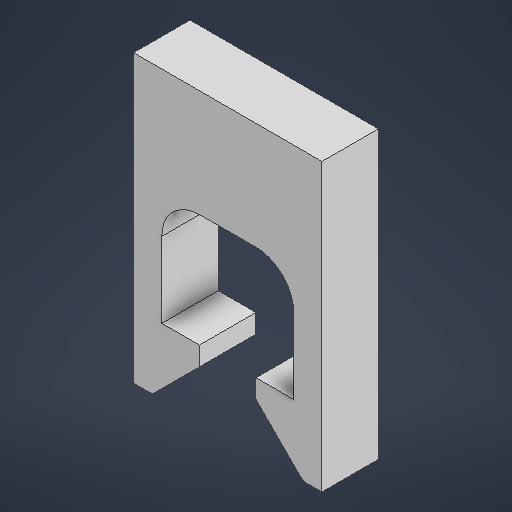
# Autodesk Inventor part: P_Wing_Mountingplate_pin
Saved by Autodesk Inventor 2026 (Build 300175000, 175)
## iProperties
Created: 2025-09-10
Part Number: P_Wing_Mountingplate_pin
Material: Generisch
Document SubType Name: Modeling
Designer: FAL
Density: 1 g/cm^3
Appearance: Vorgabe
Author: FAL
Autodesk Inventor part; units mm, degrees
ref_plane "YZ Plane" through (0, 0, 0) normal (1, 0, 0) x (0, 1, 0)
ref_plane "XZ Plane" through (0, 0, 0) normal (0, 1, 0) x (-1, 0, 0)
ref_plane "XY Plane" through (0, 0, 0) normal (0, 0, 1) x (1, 0, 0)
sketch "Skizze3" plane through (0, 0, 0) normal (0, 1, 0) x (-1, 0, 0)
  line L0 (3.5, 0) -> (3.5, -6)
  line L1 (3.5, -6) -> (1.5, -6)
  line L2 (1.5, -6) -> (1.5, -7)
  line L3 (1.5, -7) -> (4, -9.5)
  line L4 (4, -9.5) -> (5, -9.5)
  line L5 (5, -9.5) -> (5, 15)
  line L6 (5, 15) -> (0, 15)
  line L7 (0, 15) -> (0, 0)
  line L8 (0, 0) -> (3.5, 0)
  dimension "d11" = 1.5
  dimension "d12" = 6
  dimension "d13" = 1
  dimension "d14" = 1
  dimension "d15" = 45
  dimension "d16" = 2
  dimension "d17" = 5
  dimension "d18" = 15
  constraints: 18 end point, 4 perpendicular, 2 vertical, 1 coincident, 1 horizontal, 1 parallel
  measures "d11" distance between parallel lines of L0 L5
  measures "d12" distance between parallel lines of L8 L1
  measures "d13" distance of L1.end L2.end
  measures "d14" distance of L3.end L4.end
  measures "d15" angle of L0 L3
  measures "d16" distance between parallel lines of L0 L2
  measures "d17" distance between parallel lines of L7 L5
  measures "d18" distance between parallel lines of L8 L6
extrude "Extrusion2" add sketch "Skizze3" along normal blind 3
fillet "Rundung3" radius 2 1 edges at (-3.5, 1.5, 0)
mirror "Spiegeln1" about plane through (0, 0, 0) normal (1, 0, 0)
sketch "Skizze4" plane through (0, 0, 0) normal (0, -1, 0) x (1, 0, 0)
  line L0 (8.8814, 5.692) -> (-19.2057, 5.692)
  line L1 (-19.2057, 5.692) -> (-19.2057, 25.183)
  line L2 (-19.2057, 25.183) -> (8.8814, 25.183)
  line L3 (8.8814, 25.183) -> (8.8814, 5.692)
  point P0 (0, 0)
  constraints: 8 end point, 2 parallel, 1 horizontal, 1 perpendicular
extrude "Extrusion3" cut sketch "Skizze4" against normal blind 10
